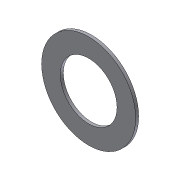
# Autodesk Inventor part: MCMASTER 90792A312
Saved by Autodesk Inventor 2014 SP1 (Build 180222100, 222)
## iProperties
Created: 2011-12-13
Part Number: MCMASTER 90792A312
Document SubType Name: Modeling
Designer: Robert Davis
Density: 8.08 g/cm^3
Material: Stainless Steel
Mass: 0.0647333 g
Surface Area: 0.732577 cm^2
Volume: 0.00801155 cm^3
Description: SHIM WASHER, 3/16" ID X 0.010"
Appearance: Steel
Author: Robert Davis
Autodesk Inventor part; units mm, degrees
ref_plane "YZ Plane" through (0, 0, 0) normal (1, 0, 0) x (0, 1, 0)
ref_plane "XZ Plane" through (0, 0, 0) normal (0, 1, 0) x (-1, 0, 0)
ref_plane "XY Plane" through (0, 0, 0) normal (0, 0, 1) x (1, 0, 0)
sketch "Sketch1" plane through (0, 0, 0) normal (0, 0, 1) x (1, 0, 0)
  circle A0 centre (0, 0) radius 2.4003
  circle A1 centre (0, 0) radius 3.9751
  dimension "d0" = 4.8006
  dimension "d1" = 7.9502
  constraints: 2 centre point
  measures "d0" diameter of A0
  measures "d1" diameter of A1
extrude "Extrusion1" add sketch "Sketch1" along normal blind 0.254
body "Solid1"
